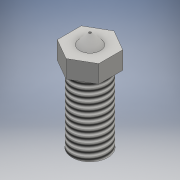
# Autodesk Inventor part: nozzle
Saved by Autodesk Inventor 2016 SP1 (Build 200210100, 210)
## iProperties
Created: 2016-04-15
Part Number: nozzle
Material: Generic
Document SubType Name: Modeling
Designer: ubik
Density: 1 g/cm^3
Appearance: Default
Author: ubik
Autodesk Inventor part; units mm, degrees
ref_plane "YZ Plane" through (0, 0, 0) normal (1, 0, 0) x (0, 1, 0)
ref_plane "XZ Plane" through (0, 0, 0) normal (0, 1, 0) x (-1, 0, 0)
sketch "Sketch1" plane through (0, 0, 0) normal (0, 0, 1) x (1, 0, 0)
  circle A0 centre (0, 0) radius 3
  dimension "d0" = 6
  constraints: 1 centre point, 1 coincident
  measures "d0" diameter of A0
extrude "Extrusion1" add sketch "Sketch1" along normal blind 12
sketch "Sketch2" plane through (0, 0, 12) normal (0, 0, 1) x (1, 0, 0)
  line L0 (3.5, -2.0207) -> (0, -4.0415)
  line L1 (0, -4.0415) -> (-3.5, -2.0207)
  line L2 (-3.5, -2.0207) -> (-3.5, 2.0207)
  line L3 (-3.5, 2.0207) -> (0, 4.0415)
  line L4 (0, 4.0415) -> (3.5, 2.0207)
  line L5 (3.5, 2.0207) -> (3.5, -2.0207)
  point P0 (0, 0)
  point P1 (0, 0)
  dimension "d3" = 7
  constraints: 12 end point, 1 coincident, 13 other
  measures "d3" distance between parallel lines of L0 L3
extrude "Extrusion2" add sketch "Sketch2" along normal blind 3
sketch "Sketch3" plane through (3.5, -2.0207, 12) normal (1, 0, 0) x (0, 0, -1)
  line L0 (12, 2.0207) -> (-9.0637, 2.0207) construction
  line L1 (-5, 2.0207) -> (-3, 3.7707)
  line L2 (-3, 0) -> (-3, 4.0415) projected
  dimension "d6" = 2
  dimension "d7" = 1.75
  constraints: 4 end point, 2 point on line, 1 horizontal
  measures "d6" distance from line of L2 L1.start
  measures "d7" distance from line of L0 L1.end
ref_plane "Work Plane1" through (0, 4.0415, 15) normal (1, 0, 0) x (0, 1, 0)
sketch "Sketch4" plane through (0, 4.0415, 15) normal (1, 0, 0) x (0, 1, 0)
  line L0 (-4.0415, -15) -> (-4.0415, 0)
  line L1 (-4.0415, 2) -> (-2.2915, 0)
  line L2 (-6.0622, 0) -> (-2.0207, 0) projected
  line L3 (-4.0415, 2) -> (-4.0415, 9.3092)
  line L4 (-4.0415, 0) -> (-4.0415, 2)
  line L5 (-2.2915, 0) -> (-4.0415, 0)
  dimension "d8" = 1.75
  dimension "d9" = 2
  constraints: 10 end point, 3 vertical, 1 collinear, 1 midpoint, 1 point on line
  measures "d8" distance from line of L0 L1.end
  measures "d9" distance from line of L2 L1.start
revolve "Revolution1" add sketch "Sketch4" angle 360 about axis through (0, 0, 17) along (0, 0, 1)
sketch "Sketch5" plane through (0, 0, 0) normal (0, 0, -1) x (-1, 0, 0)
  circle A0 centre (0, 0) radius 0.875
  dimension "d11" = 1.75
  constraints: 1 centre point, 1 coincident
  measures "d11" diameter of A0
extrude "Extrusion3" cut sketch "Sketch5" against normal blind 15
sketch "Sketch6" plane through (0, 0, 15) normal (0, 0, -1) x (-1, 0, 0)
  circle A0 centre (0, 0) radius 0.2
  dimension "d14" = 0.4
  constraints: 1 centre point, 1 coincident
  measures "d14" diameter of A0
extrude "Extrusion4" cut sketch "Sketch6" against normal through all
thread "Thread1" size "M6x1" class "6g" standard "ANSI Metric M Profile" full length
body "Solid1"
